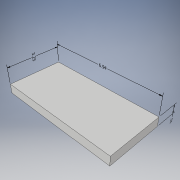
# Autodesk Inventor part: Part_A
Saved by Autodesk Inventor 2019 (Build 230136000, 136)
## iProperties
Created: 2018-12-29
Part Number: Part_A
Material: Generic
Document SubType Name: Modeling
Designer: Owner
Density: 1 g/cm^3
Appearance: Default
Author: Owner
Autodesk Inventor part; units mm, degrees
ref_plane "YZ Plane" through (0, 0, 0) normal (1, 0, 0) x (0, 1, 0)
ref_plane "XZ Plane" through (0, 0, 0) normal (0, 1, 0) x (-1, 0, 0)
ref_plane "XY Plane" through (0, 0, 0) normal (0, 0, 1) x (1, 0, 0)
sketch "Sketch1" plane through (0, 0, 0) normal (0, 1, 0) x (-1, 0, 0)
  line L0 (0, 0) -> (6.6211, 0)
  line L1 (0, 0) -> (176.2125, 0)
  line L2 (176.2125, 0) -> (176.2125, -82.55)
  line L3 (176.2125, -82.55) -> (0, -82.55)
  line L4 (0, -82.55) -> (0, 0)
  dimension "d0" = 176.2125
  dimension "d1" = 82.55
  constraints: 10 end point, 2 horizontal, 2 parallel, 1 perpendicular, 1 point on line
  measures "d0" distance of L2.end L3.end
  measures "d1" distance of L1.end L2.end
extrude "Extrusion1" add sketch "Sketch1" along normal blind 14.2875
body "Solid1"
